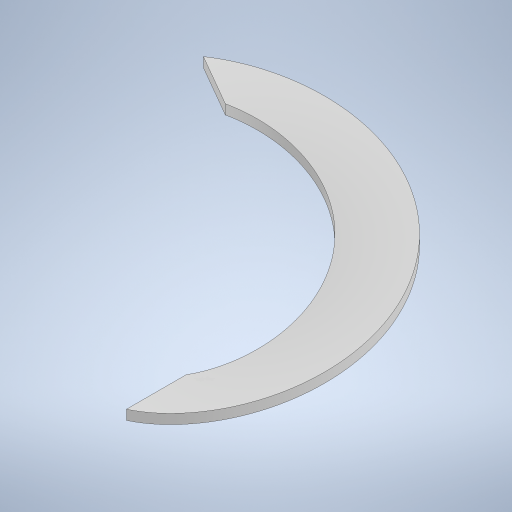
# Autodesk Inventor part: Espira_01_Parcial
Saved by Autodesk Inventor 2024 (Build 280153000, 153)
## iProperties
Created: 2026-01-07
Part Number: Espira_01_Parcial
Material: Generic
Document SubType Name: Modeling
Designer: eduso
Density: 1 g/cm^3
Appearance: Default
Paso_Espira_01: 150.000 mm
ø_Ext_Espira_01: 150.000 mm
ø_Int_Espira_01: 76.100 mm
Espesor_Espira_01: 6.000 mm
Author: eduso
Autodesk Inventor part; units mm, degrees
ref_plane "YZ Plane" through (0, 0, 0) normal (1, 0, 0) x (0, 1, 0)
ref_plane "XY Plane" through (0, 0, 0) normal (0, 0, 1) x (1, 0, 0)
sketch "Sketch1" plane through (0, 0, 0) normal (0, 1, 0) x (-1, 0, 0)
  circle A0 centre (0, 0) radius 38.05 construction
  line L0 (0, 0) -> (0, 38.05) construction
  dimension "d0" = 76.1
  constraints: 2 end point, 1 coincident, 1 vertical, 1 vertical alignment, 2 other
ref_plane "Work Plane1" through (0, 6, 0) normal (0, 1, 0) x (-1, 0, 0)
sketch "Sketch2" plane through (0, 6, 0) normal (0, 1, 0) x (-1, 0, 0)
  circle A0 centre (0, 0) radius 75 construction
  line L0 (0, 0) -> (0, 75) construction
  dimension "d2" = 150
  constraints: 2 end point, 1 coincident, 1 vertical, 1 vertical alignment, 2 other
sketch "Sketch3" plane through (0, 0, 0) normal (1, 0, 0) x (0, 1, 0)
  line L0 (0, 38.05) -> (6, 38.05)
  line L1 (6, 38.05) -> (6, 75)
  line L2 (6, 75) -> (0, 75)
  line L3 (0, 75) -> (0, 38.05)
  line L4 (0, 0) -> (150, 0) construction
  line L5 (0, 0) -> (0, 38.05)
  line L6 (6, 75) -> (6, 0) construction
  dimension "d3" = 150
  dimension "d12" = 38.05
  dimension "d13" = 75
  dimension "d14" = 6
  constraints: 14 end point, 2 horizontal, 2 parallel, 2 vertical, 1 perpendicular, 1 point on line
  measures "d3" distance of L4.start L4.end
  measures "d12" distance of L4.start L0.start
  measures "d13" distance of L1.end L6.end
  measures "d14" distance of L1.end L2.end
coil "Coil1" sketch "Sketch3" operation add axis through (0, 0, 0) along (0, 1, 0) pitch 150 turns 0.666667 hand right
equation "\"d0\" = ø_Int_Espira_01"
equation "\"d2\" = ø_Ext_Espira_01"
equation "\"d12\" = 0.5 * ø_Int_Espira_01"
equation "\"d13\" = 0.5 * ø_Ext_Espira_01"
equation "\"d14\" = Espesor_Espira_01"
equation "\"d6\" = Ang_parcial"
equation "\"ø_Ext_Espira_01\" = 150"
equation "\"ø_Int_Espira_01\" = 76.1"
equation "\"Espesor_Espira_01\" = 6"
equation "\"d1\" = Espesor_Espira_01"
equation "\"L_parcial\" = 276.66667"
equation "\"Ang_parcial\" = 0.666667"
body "Solid1"
